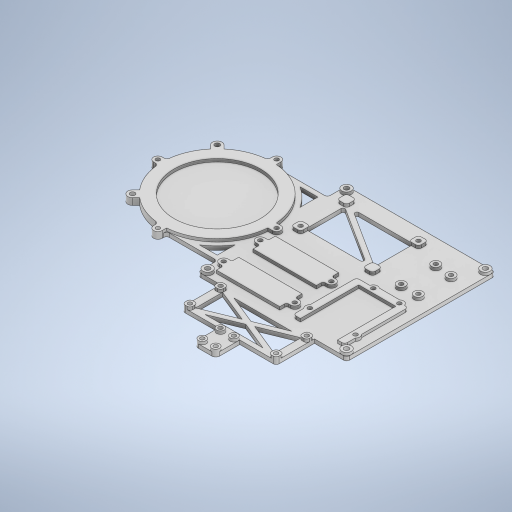
# Autodesk Inventor part: Base_BasePlate
Saved by Autodesk Inventor 2023 (Build 270158000, 158)
## iProperties
Created: 2025-02-05
Part Number: Base_BasePlate
Material: Generic
Document SubType Name: Modeling
Designer: Swoby
Density: 1 g/cm^3
Appearance: Default
Author: Swoby
Autodesk Inventor part; units mm, degrees
ref_plane "YZ Plane" through (0, 0, 0) normal (1, 0, 0) x (0, 1, 0)
ref_plane "XZ Plane" through (0, 0, 0) normal (0, 1, 0) x (-1, 0, 0)
ref_plane "XY Plane" through (0, 0, 0) normal (0, 0, 1) x (1, 0, 0)
sketch "Sketch1" plane through (0, 0, 0) normal (0, 1, 0) x (-1, 0, 0)
  line L0 (77.5, 77.5) -> (-77.5, 77.5)
  line L1 (-77.5, 77.5) -> (-77.5, -77.5)
  line L2 (-77.5, -77.5) -> (77.5, -77.5)
  line L3 (77.5, -77.5) -> (77.5, 77.5) construction
  line L4 (77.5, 77.5) -> (-77.5, -77.5) construction
  line L5 (-77.5, 77.5) -> (77.5, -77.5) construction
  line L6 (67.5, -9.5) -> (-17.6, -9.5) construction
  line L7 (-17.6, -9.5) -> (-17.6, -67.5) construction
  line L8 (-17.6, -67.5) -> (67.5, -67.5) construction
  line L9 (67.5, -67.5) -> (67.5, -9.5) construction
  line L10 (67.5, -9.5) -> (-17.6, -67.5) construction
  line L11 (-17.6, -9.5) -> (67.5, -67.5) construction
  circle A0 centre (62.5, -14.5) radius 2.1
  circle A1 centre (-12.6, -62.5) radius 2.1
  line L12 (57.5, -19.5) -> (67.5, -19.5)
  line L13 (67.5, -19.5) -> (67.5, -9.5)
  line L14 (67.5, -9.5) -> (57.5, -9.5)
  line L15 (57.5, -9.5) -> (57.5, -19.5)
  line L16 (57.5, -19.5) -> (67.5, -9.5) construction
  line L17 (67.5, -19.5) -> (57.5, -9.5) construction
  line L18 (-7.6, -57.5) -> (-17.6, -57.5)
  line L19 (-17.6, -57.5) -> (-17.6, -67.5)
  line L20 (-17.6, -67.5) -> (-7.6, -67.5)
  line L21 (-7.6, -67.5) -> (-7.6, -57.5)
  line L22 (-7.6, -57.5) -> (-17.6, -67.5) construction
  line L23 (-17.6, -57.5) -> (-7.6, -67.5) construction
  line L24 (-17.6, -9.5) -> (-7.6, -9.5)
  line L25 (-7.6, -9.5) -> (-7.6, -19.5)
  line L26 (-7.6, -19.5) -> (-17.6, -19.5)
  line L27 (-17.6, -19.5) -> (-17.6, -9.5)
  line L28 (67.5, -67.5) -> (57.5, -67.5)
  line L29 (57.5, -67.5) -> (57.5, -57.5)
  line L30 (57.5, -57.5) -> (67.5, -57.5)
  line L31 (67.5, -57.5) -> (67.5, -67.5)
  circle A2 centre (-42.6, -14.5) radius 2.1
  circle A3 centre (-42.6, -50.6) radius 2.1
  circle A4 centre (-60.5, -14.5) radius 2.1
  circle A5 centre (-60.5, -48.6) radius 2.1
  line L32 (-42.6, -14.5) -> (-42.6, -50.6) construction
  line L33 (-42.6, -14.5) -> (-60.5, -14.5) construction
  line L34 (-60.5, -14.5) -> (-60.5, -48.6) construction
  circle A6 centre (-42.6, -14.5) radius 4.5
  circle A7 centre (-42.6, -50.6) radius 4.5
  circle A8 centre (-60.5, -14.5) radius 4.5
  circle A9 centre (-60.5, -48.6) radius 4.5
  line L35 (-13.8, 69.5) -> (-67.5, 69.5)
  line L36 (-67.5, 69.5) -> (-67.5, 3.2)
  line L37 (-13.8, 3.2) -> (-13.8, 69.5)
  line L38 (-63.9, 3.2) -> (-61.4, 0.7)
  line L39 (-61.4, 0.7) -> (-29.8, 0.7)
  line L40 (-29.8, 0.7) -> (-27.3, 3.2)
  line L41 (-67.5, 3.2) -> (-63.9, 3.2)
  line L42 (-27.3, 3.2) -> (-13.8, 3.2)
  circle A10 centre (-64.5, 55.1) radius 2.1
  circle A11 centre (-16.8, 55.1) radius 2.1
  line L43 (77.5, 0) -> (77.5, 77.5) construction
  line L44 (77.5, 38.75) -> (5.2514, 38.75) construction
  line L45 (66.4, 69.5) -> (0.2, 69.5)
  line L46 (0.2, 69.5) -> (0.2, 62.35)
  line L47 (0.2, 46.2) -> (66.4, 46.2)
  line L48 (66.4, 46.2) -> (66.4, 69.5)
  circle A12 centre (-3.8, 57.85) radius 2.1
  circle A13 centre (70.4, 57.85) radius 2.1
  arc A14 (70.4, 53.35) -> (70.4, 62.35) centre (70.4, 57.85) ccw
  arc A15 (-3.8, 62.35) -> (-3.8, 53.35) centre (-3.8, 57.85) ccw
  line L49 (-3.8, 62.35) -> (0.2, 62.35)
  line L50 (-3.8, 53.35) -> (0.2, 53.35)
  line L51 (70.4, 62.35) -> (66.4, 62.35)
  line L52 (70.4, 53.35) -> (66.4, 53.35)
  line L53 (-3.8, 57.85) -> (70.4, 57.85) construction
  line L54 (33.3, 69.5) -> (33.3, 46.2) construction
  line L55 (66.4, 8) -> (0.2, 8)
  line L56 (0.2, 8) -> (0.2, 15.15)
  line L57 (0.2, 31.3) -> (66.4, 31.3)
  line L58 (66.4, 31.3) -> (66.4, 24.15)
  circle A16 centre (-3.8, 19.65) radius 2.1
  circle A17 centre (70.4, 19.65) radius 2.1
  arc A18 (70.4, 15.15) -> (70.4, 24.15) centre (70.4, 19.65) ccw
  arc A19 (-3.8, 24.15) -> (-3.8, 15.15) centre (-3.8, 19.65) ccw
  line L59 (-3.8, 15.15) -> (0.2, 15.15)
  line L60 (-3.8, 24.15) -> (0.2, 24.15)
  line L61 (70.4, 15.15) -> (66.4, 15.15)
  line L62 (70.4, 24.15) -> (66.4, 24.15)
  line L63 (-3.8, 19.65) -> (70.4, 19.65) construction
  line L64 (33.3, 8) -> (33.3, 31.3) construction
  circle A20 centre (-32, 4.1) radius 2.1
  circle A21 centre (-59.2, 4.1) radius 2.1
  line L65 (-32, 4.1) -> (-59.2, 4.1) construction
  line L66 (54, 117.5) -> (-44, 117.5)
  line L67 (-44, 117.5) -> (-44, 77.5)
  line L68 (-44, 77.5) -> (54, 77.5) construction
  line L69 (54, 77.5) -> (54, 117.5)
  line L70 (54, 117.5) -> (-44, 77.5) construction
  line L71 (-44, 117.5) -> (54, 77.5) construction
  line L72 (35.1344, 112.5) -> (-25.1344, 112.5)
  line L73 (-25.1344, 112.5) -> (5, 100.2002)
  line L74 (5, 100.2002) -> (35.1344, 112.5)
  line L75 (46, 111.5345) -> (11.6156, 97.5)
  line L76 (11.6156, 97.5) -> (46, 83.4655)
  line L77 (46, 83.4655) -> (46, 111.5345)
  line L78 (-36, 111.5345) -> (-1.6156, 97.5)
  line L79 (-1.6156, 97.5) -> (-36, 83.4655)
  line L80 (-36, 83.4655) -> (-36, 111.5345)
  line L81 (5, 94.7998) -> (-25.1344, 82.5)
  line L82 (-25.1344, 82.5) -> (35.1344, 82.5)
  line L83 (35.1344, 82.5) -> (5, 94.7998)
  line L84 (-40, 113.5) -> (50, 113.5) construction
  line L85 (50, 113.5) -> (50, 81.5) construction
  line L86 (50, 81.5) -> (-40, 81.5) construction
  line L87 (-40, 81.5) -> (-40, 113.5) construction
  line L88 (-40, 113.5) -> (50, 81.5) construction
  line L89 (50, 113.5) -> (-40, 81.5) construction
  circle A22 centre (50, 113.5) radius 2.1
  circle A23 centre (50, 81.5) radius 2.1
  circle A24 centre (-40, 113.5) radius 2.1
  circle A25 centre (-40, 81.5) radius 2.1
  line L90 (46, 109.5) -> (54, 109.5)
  line L91 (54, 109.5) -> (54, 117.5)
  line L92 (54, 117.5) -> (46, 117.5)
  line L93 (46, 117.5) -> (46, 109.5)
  line L94 (46, 109.5) -> (54, 117.5) construction
  line L95 (54, 109.5) -> (46, 117.5) construction
  line L96 (46, 85.5) -> (54, 85.5)
  line L97 (54, 85.5) -> (54, 77.5)
  line L98 (54, 77.5) -> (46, 77.5)
  line L99 (46, 77.5) -> (46, 85.5)
  line L100 (46, 85.5) -> (54, 77.5) construction
  line L101 (54, 85.5) -> (46, 77.5) construction
  line L102 (-36, 85.5) -> (-44, 85.5)
  line L103 (-44, 85.5) -> (-44, 77.5)
  line L104 (-44, 77.5) -> (-36, 77.5)
  line L105 (-36, 77.5) -> (-36, 85.5)
  line L106 (-36, 85.5) -> (-44, 77.5) construction
  line L107 (-44, 85.5) -> (-36, 77.5) construction
  line L108 (-36, 109.5) -> (-44, 109.5)
  line L109 (-44, 109.5) -> (-44, 117.5)
  line L110 (-44, 117.5) -> (-36, 117.5)
  line L111 (-36, 117.5) -> (-36, 109.5)
  line L112 (-36, 109.5) -> (-44, 117.5) construction
  line L113 (-44, 109.5) -> (-36, 117.5) construction
  circle A26 centre (135, 0) radius 45
  line L114 (135, 0) -> (77.5, 0) construction
  circle A27 centre (135, 0) radius 57.5
  line L115 (135, 57.5) -> (130.5, 57.5) construction
  line L116 (135, -57.5) -> (130.5, -57.5) construction
  line L117 (101.0884, 52.5) -> (82.5, 52.5)
  line L118 (82.5, 52.5) -> (82.5, 33.9116)
  arc A28 (101.0884, 52.5) -> (82.5, 33.9116) centre (135, 0) ccw
  line L119 (101.0884, -52.5) -> (82.5, -52.5)
  line L120 (82.5, -52.5) -> (82.5, -33.9116)
  arc A29 (82.5, -33.9116) -> (101.0884, -52.5) centre (135, 0) ccw
  arc A30 (77.5, 0) -> (73, 4.5) centre (73, 0) ccw construction
  circle A31 centre (73, 0) radius 2.1
  line L121 (135, 0) -> (192.5, 0) construction
  line L122 (135, 57.5) -> (135, -57.5) construction
  arc A32 (197, -4.5) -> (197, 4.5) centre (197, 0) ccw
  circle A33 centre (197, 0) radius 2.1
  line L123 (197, 4.5) -> (192.3236, 4.5)
  line L124 (197, -4.5) -> (192.3236, -4.5)
  line L125 (73, 4.5) -> (77.6764, 4.5)
  line L126 (73, -4.5) -> (77.6764, -4.5)
  line L127 (77.5, 77.5) -> (77.5, 57.5)
  line L128 (77.5, -77.5) -> (77.5, -57.5)
  arc A34 (139.5, 62) -> (130.5, 62) centre (135, 62) ccw
  circle A35 centre (135, 62) radius 2.1
  line L129 (139.5, 62) -> (139.5, 57.3236)
  line L130 (130.5, 62) -> (130.5, 57.3236)
  arc A36 (130.5, -62) -> (139.5, -62) centre (135, -62) ccw
  circle A37 centre (135, -62) radius 2.1
  line L131 (130.5, -62) -> (130.5, -57.3236)
  line L132 (139.5, -62) -> (139.5, -57.3236)
  line L133 (5, 97.5) -> (5, 117.5) construction
  circle A38 centre (-16.8, 55.1) radius 4.5
  circle A39 centre (-64.5, 55.1) radius 4.5
  circle A40 centre (-32, 4.1) radius 4.5
  circle A41 centre (-59.2, 4.1) radius 4.5
  line L134 (-21.3, 69.5) -> (-21.3, 8.6)
  line L135 (-21.3, 8.6) -> (-60, 8.6)
  line L136 (-60, 8.6) -> (-60, 69.5)
  arc A42 (73, -4.5) -> (77.5, 0) centre (73, 0) ccw construction
  arc A43 (73, 4.5) -> (73, -4.5) centre (73, 0) ccw
  line L137 (130.5, 57.5) -> (77.5, 57.5)
  line L138 (130.5, -57.5) -> (77.5, -57.5)
  line L139 (66.4, 15.15) -> (66.4, 8)
  line L140 (66.4, 19.65) -> (66.4, 15.15) construction
  line L141 (66.4, 24.15) -> (66.4, 19.65) construction
  line L142 (0.2, 15.15) -> (0.2, 24.15) construction
  line L143 (0.2, 24.15) -> (0.2, 31.3)
  line L144 (0.2, 62.35) -> (0.2, 53.35) construction
  line L145 (0.2, 53.35) -> (0.2, 46.2)
  point P0 (0, 0)
  point P1 (24.95, -38.5)
  point P2 (-51.55, -14.5)
  point P3 (-77.5, 0)
  point P4 (66.4, 57.85)
  point P5 (33.3, 57.85)
  point P6 (-8.3, 57.85)
  point P7 (33.3, 19.65)
  point P8 (-8.3, 19.65)
  point P9 (-67.5, 58.4541)
  point P10 (-67.5, 51.7459)
  point P11 (-63.5116, 2.8116)
  point P12 (-56.2521, 0.7)
  point P13 (-34.9479, 0.7)
  point P14 (-27.6884, 2.8116)
  point P15 (-13.8, 51.7459)
  point P16 (-13.8, 58.4541)
  dimension "d99" = 115
  dimension "d0" = 155
  dimension "d1" = 155
  dimension "d2" = 85.1
  dimension "d3" = 58
  dimension "d5" = 10
  dimension "d6" = 4.2
  dimension "d7" = 4.2
  dimension "d8" = 5
  dimension "d9" = 5
  dimension "d10" = 5
  dimension "d11" = 5
  dimension "d14" = 10
  dimension "d15" = 10
  dimension "d16" = 10
  dimension "d17" = 10
  dimension "d18" = 10
  dimension "d21" = 4.2
  dimension "d22" = 4.2
  dimension "d23" = 4.2
  dimension "d24" = 4.2
  dimension "d25" = 17.9
  dimension "d26" = 17.9
  dimension "d27" = 25
  dimension "d28" = 5
  dimension "d29" = 36.1
  dimension "d30" = 34.1
  dimension "d31" = 9
  dimension "d32" = 9
  dimension "d33" = 9
  dimension "d34" = 9
  dimension "d35" = 66.3
  dimension "d36" = 53.7
  dimension "d39" = 10
  dimension "d40" = 31.6
  dimension "d43" = 13.5
  dimension "d44" = 135
  dimension "d45" = 135
  dimension "d46" = 2.5
  dimension "d47" = 3
  dimension "d48" = 14.4
  dimension "d49" = 4.2
  dimension "d50" = 4.2
  dimension "d51" = 3
  dimension "d52" = 14.4
  dimension "d53" = 4.2
  dimension "d54" = 4.2
  dimension "d55" = 9
  dimension "d56" = 9
  dimension "d58" = 66.2
  dimension "d59" = 74.2
  dimension "d62" = 23.3
  dimension "d63" = 14
  dimension "d64" = 4.2
  dimension "d65" = 4.2
  dimension "d66" = 27.2
  dimension "d67" = 3.4
  dimension "d68" = 8.3
  dimension "d72" = 8
  dimension "d73" = 40
  dimension "d74" = 98
  dimension "d75" = 23.5
  dimension "d76" = 5
  dimension "d78" = 2.5
  dimension "d80" = 2.5
  constraints: 292 end point, 48 parallel, 43 centre point, 32 perpendicular, 30 midpoint, 27 horizontal, 25 point on circle, 25 point on line, 24 symmetric about line, 21 coincident, 21 tangent, 8 vertical, 4 collinear, 20 other
  measures "d0" distance of L2.end L1.end
  measures "d1" distance of L1.end L0.end
  measures "d2" distance of L8.end L7.end
  measures "d3" distance of L7.end L6.end
  measures "d5" distance between parallel lines of L3 L9
  measures "d6" diameter of A0
  measures "d7" diameter of A1
  measures "d8" distance from line of L9 A0.centre
  measures "d9" distance from line of L6 A0.centre
  measures "d10" distance from line of L7 A1.centre
  measures "d11" distance from line of L8 A1.centre
  measures "d14" distance between parallel lines of L2 L8
  measures "d15" distance of L25.end L26.end
  measures "d16" distance of L24.end L25.end
  measures "d17" distance of L29.end L30.end
  measures "d18" distance of L28.end L29.end
  measures "d21" diameter of A2
  measures "d22" diameter of A3
  measures "d23" diameter of A4
  measures "d24" diameter of A5
  measures "d25" distance of L32.start L33.end
  measures "d26" horizontal distance of L34.end L32.end
  measures "d27" distance between parallel lines of L32 L7
  measures "d28" distance from line of point (-51.55, -14.5) L6
  measures "d29" distance of L32.start L32.end
  measures "d30" distance of L33.end L34.end
  measures "d31" diameter of A6
  measures "d32" diameter of A7
  measures "d33" diameter of A8
  measures "d34" diameter of A9
  measures "d35" distance of L35.end L36.end
  measures "d36" distance of L35.start L35.end
  measures "d39" distance between parallel lines of L1 L36
  measures "d40" distance of L38.end L39.end
  measures "d43" distance of L40.end L37.start
  measures "d44" angle of L40 L42
  measures "d45" angle of L41 L38
  measures "d46" distance between parallel lines of L41 L39
  measures "d47" distance from line of L36 A10.centre
  measures "d48" distance from line of L35 A10.centre
  measures "d49" diameter of A10
  measures "d50" diameter of A11
  measures "d51" distance from line of L37 A11.centre
  measures "d52" distance from line of L35 A11.centre
  measures "d53" diameter of A12
  measures "d54" diameter of A13
  measures "d55" diameter of A14
  measures "d56" diameter of A15
  measures "d58" distance of L45.start L45.end
  measures "d59" distance of L53.start L53.end
  measures "d62" distance of L47.end L45.start
  measures "d63" distance between parallel lines of L37 L46
  measures "d64" diameter of A20
  measures "d65" diameter of A21
  measures "d66" distance of L65.start L65.end
  measures "d67" distance between parallel lines of L39 L65
  measures "d68" distance from line of L36 L65.end
  measures "d72" distance between parallel lines of L0 L35
  measures "d73" distance of L66.end L67.end
  measures "d74" distance of L66.start L66.end
  measures "d75" distance between parallel lines of L69 L3
  measures "d76" distance between parallel lines of L72 L66
  measures "d78" distance between parallel lines of L70 L74
  measures "d80" distance between parallel lines of L71 L73
extrude "Extrusion1" add sketch "Sketch1" against normal blind 4 contours L127 L137 L130 A27 L125 A43 L126 L131 L138 L128 L2 L1 L0 | L0 L99 L77 L96 L69 | L0 L105 L79 L78 L111 L66 L93 L75 L76 L99 | L96 L77 L90 L69 | L130 A34 L129 A27 | L0 L67 L102 L80 L105 | L90 L77 L93 L66 L69 | A27 | A27 L126 A43 L125 | L67 L108 L80 L102 | L123 A32 L124 A27 | L67 L66 L111 L80 L108 | A27 L132 A36 L131 | A0 | A1 | L15 L14 L13 L12 | L21 L20 L19 L18 | L24 L25 L26 L27 | L28 L29 L30 L31 | A2 | A3 | A4 | A5 | A6 | A7 | A8 | A9 | L37 A38 L134 L35 | L134 L135 L136 L35 | A38 L37 | L37 A38 | L136 A39 L36 L35 | A38 L37 L42 L40 A40 L135 L134 | A39 L36 | L136 L135 A41 L38 L41 L36 A39 | L36 A39 | A40 L40 L39 | A40 L39 A41 L135 | A41 L39 L38 | L39 L40 A40 | L38 L39 A41 | A10 | A11 | L48 L47 L145 L50 A15 L49 L46 L45 | L51 A14 L52 L48 | A12 | L55 L56 L59 A19 L60 L143 L57 L58 L62 A18 L61 L139 | A16 | A17 | A20 | A21 | A23 | A25 | A26 | A31 | A33 | A35 | A37
extrude "Extrusion2" add sketch "Sketch1" along normal blind 3 contours L0 L99 L77 L96 L69 | L130 A34 L129 A27 | L0 L67 L102 L80 L105 | L90 L77 L93 L66 L69 | A27 | A27 L126 A43 L125 | L123 A32 L124 A27 | L67 L66 L111 L80 L108 | A27 L132 A36 L131 | L15 L14 L13 L12 | L21 L20 L19 L18 | L24 L25 L26 L27 | L28 L29 L30 L31 | A6 | A7 | A8 | A9 | L37 A38 L134 L35 | A38 L37 | L37 A38 | L136 A39 L36 L35 | A38 L37 L42 L40 A40 L135 L134 | A39 L36 | L136 L135 A41 L38 L41 L36 A39 | L36 A39 | A40 L40 L39 | A40 L39 A41 L135 | A41 L39 L38 | L39 L40 A40 | L38 L39 A41 | L48 L47 L145 L50 A15 L49 L46 L45 | L51 A14 L52 L48 | L55 L56 L59 A19 L60 L143 L57 L58 L62 A18 L61 L139
fillet "Fillet1" radius 2 8 edges at (-0.2, 1.5, 53.35) (-0.2, 1.5, 62.35) (-0.2, 1.5, 24.15) (-0.2, 1.5, 15.15) (-66.4, 1.5, 62.35) (-66.4, 1.5, 53.35) (-66.4, 1.5, 24.15) (-66.4, 1.5, 15.15)
extrude "Extrusion3" cut sketch "Sketch1" against normal through all contours A0 | A1 | A2 | A5 | A10 | A11 | A12 | A13 | A16 | A17 | A20 | A21 | A22 | A23 | A24 | A25 | A31 | A33 | A35 | A37
fillet "Fillet2" radius 3 50 edges at (44, 1.5, 109.5) (36, 1.5, 109.5) (36, 1.5, 117.5) (67.5, 1.5, 69.5) (44, 1.5, 85.5) (36, 1.5, 85.5) (36, 1.5, 77.5) (44, 1.5, 77.5) (-54, 1.5, 109.5) (-46, 1.5, 117.5) (-46, 1.5, 109.5) (-46, 1.5, 85.5) (-46, 1.5, 77.5) (-54, 1.5, 77.5) (-54, 1.5, 85.5) (67.5, 1.5, 3.2) (13.8, 1.5, 3.2) (13.8, 1.5, 69.5) (17.6, 1.5, -9.5) (7.6, 1.5, -9.5) (7.6, 1.5, -19.5) (17.6, 1.5, -19.5) (7.6, 1.5, -57.5) (7.6, 1.5, -67.5) (17.6, 1.5, -57.5) (17.6, 1.5, -67.5) (-67.5, 1.5, -9.5) (-67.5, 1.5, -19.5) (-57.5, 1.5, -9.5) (-57.5, 1.5, -19.5) (-67.5, 1.5, -67.5) (-67.5, 1.5, -57.5) (-57.5, 1.5, -57.5) (-57.5, 1.5, -67.5) (-130.5, -2, 57.5) (-77.5, -2, 57.5) (-77.5, -2, -57.5) (-130.5, -2, -57.5) (-139.5, -0.5, -57.3236) (-139.5, -2, 57.3236) (-139.5, 1.5, 57.3236) (-192.3236, -2, 4.5) (-192.3236, 1.5, 4.5) (-192.3236, -0.5, -4.5) (-54, -0.5, 117.5) (44, -0.5, 117.5) (-77.5, -2, 77.5) (-77.5, -2, -77.5) (77.5, -2, -77.5) (77.5, -2, 77.5)
sketch "Sketch2" plane through (0, 0, 0) normal (0, 1, 0) x (1, 0, 0)
  circle A0 centre (-62.5, 14.5) radius 2.1 projected
  circle A1 centre (12.6, 62.5) radius 2.1 projected
  line L0 (-62.5, 14.5) -> (5.7571, 14.5) construction
  line L1 (12.6, 18.1519) -> (12.6, 62.5) construction
  line L2 (12.6, 62.5) -> (-55.6571, 62.5) construction
  line L3 (-62.5, 58.8481) -> (-62.5, 14.5) construction
  line L4 (-59.4229, 60.5333) -> (6.8342, 18.1852) construction
  line L5 (-56.7342, 58.8148) -> (9.5229, 16.4667) construction
  arc A2 (-59.4229, 60.5333) -> (-62.5, 58.8481) centre (-60.5, 58.8481) ccw construction
  arc A3 (-55.6571, 62.5) -> (-56.7342, 58.8148) centre (-55.6571, 60.5) ccw construction
  arc A4 (5.7571, 14.5) -> (6.8342, 18.1852) centre (5.7571, 16.5) ccw
  arc A5 (9.5229, 16.4667) -> (12.6, 18.1519) centre (10.6, 18.1519) ccw
  line L6 (-57.542, 17) -> (-2.7965, 17)
  line L7 (-1.7194, 20.6852) -> (-56.9229, 55.9684)
  line L8 (-60, 54.2832) -> (-60, 19.458)
  line L9 (-47.1035, 60) -> (7.642, 60)
  line L10 (10.1, 57.542) -> (10.1, 22.7168)
  line L11 (7.0229, 21.0316) -> (-48.1806, 56.3148)
  arc A6 (-56.9229, 55.9684) -> (-60, 54.2832) centre (-58, 54.2832) ccw
  arc A7 (-2.7965, 17) -> (-1.7194, 20.6852) centre (-2.7965, 19) ccw
  arc A8 (7.0229, 21.0316) -> (10.1, 22.7168) centre (8.1, 22.7168) ccw
  arc A9 (-47.1035, 60) -> (-48.1806, 56.3148) centre (-47.1035, 58) ccw
  arc A10 (-57.5, 16.5) -> (-60.5, 19.5) centre (-60.5, 16.5) ccw projected
  arc A11 (7.6, 60.5) -> (10.6, 57.5) centre (10.6, 60.5) ccw projected
  point P0 (0, 0)
  point P1 (12.6, 14.5)
  point P2 (-62.5, 62.5)
  dimension "d115" = 2
  dimension "d116" = 2
  dimension "d117" = 2.5
  dimension "d118" = 2.5
  dimension "d119" = 2
  dimension "d120" = 2.5
  dimension "d121" = 2.5
  dimension "d122" = 2.5
  dimension "d123" = 2.5
  constraints: 24 end point, 20 point on circle, 16 tangent, 8 centre point, 8 point on line, 6 parallel, 5 equal radius, 1 horizontal, 1 perpendicular
  measures "d115" radius of A2
  measures "d116" radius of A3
  measures "d117" distance between parallel lines of L3 L8
  measures "d118" distance between parallel lines of L2 L9
  measures "d119" radius of A6
  measures "d120" distance between parallel lines of L5 L7
  measures "d121" distance between parallel lines of L11 L4
  measures "d122" distance between parallel lines of L0 L6
  measures "d123" distance between parallel lines of L1 L10
extrude "Extrusion5" cut sketch "Sketch2" against normal through all contours A10 L8 A6 L7 A7 L6 | L9 A11 L10 A8 L11 A9
sketch "Sketch3" plane through (0, 0, 0) normal (0, 1, 0) x (1, 0, 0)
  line L0 (-46, -83.4655) -> (-11.6156, -97.5) projected
  line L1 (-11.6156, -97.5) -> (-46, -111.5345) projected
  line L2 (-46, -111.5345) -> (-46, -83.4655) projected
  line L3 (36, -83.4655) -> (36, -111.5345) projected
  line L4 (36, -111.5345) -> (1.6156, -97.5) projected
  line L5 (1.6156, -97.5) -> (36, -83.4655) projected
  line L6 (-5, -94.7998) -> (-35.1344, -82.5) projected
  line L7 (-35.1344, -82.5) -> (25.1344, -82.5) projected
  line L8 (25.1344, -82.5) -> (-5, -94.7998) projected
  line L9 (-35.1344, -112.5) -> (-5, -100.2002) projected
  line L10 (-5, -100.2002) -> (25.1344, -112.5) projected
  line L11 (25.1344, -112.5) -> (-35.1344, -112.5) projected
  arc A0 (-49, -85.5) -> (-46, -82.5) centre (-49, -82.5) ccw projected
  line L12 (-49, -85.5) -> (-51, -85.5) projected
  arc A1 (-54, -82.5) -> (-51, -85.5) centre (-51, -82.5) ccw projected
  line L13 (-54, -82.5) -> (-54, -112.5) projected
  arc A2 (-51, -109.5) -> (-54, -112.5) centre (-51, -112.5) ccw projected
  line L14 (-51, -109.5) -> (-49, -109.5) projected
  arc A3 (-46, -112.5) -> (-49, -109.5) centre (-49, -112.5) ccw projected
  line L15 (-46, -112.5) -> (-46, -114.5) projected
  arc A4 (-49, -117.5) -> (-46, -114.5) centre (-49, -114.5) ccw projected
  line L16 (-49, -117.5) -> (39, -117.5) projected
  arc A5 (36, -114.5) -> (39, -117.5) centre (39, -114.5) ccw projected
  line L17 (36, -114.5) -> (36, -112.5) projected
  arc A6 (39, -109.5) -> (36, -112.5) centre (39, -112.5) ccw projected
  line L18 (39, -109.5) -> (41, -109.5) projected
  arc A7 (44, -112.5) -> (41, -109.5) centre (41, -112.5) ccw projected
  line L19 (44, -112.5) -> (44, -82.5) projected
  arc A8 (41, -85.5) -> (44, -82.5) centre (41, -82.5) ccw projected
  line L20 (41, -85.5) -> (39, -85.5) projected
  arc A9 (36, -82.5) -> (39, -85.5) centre (39, -82.5) ccw projected
  line L21 (36, -82.5) -> (36, -80.5) projected
  arc A10 (39, -77.5) -> (36, -80.5) centre (39, -80.5) ccw projected
  line L22 (39, -77.5) -> (41, -77.5) projected
  arc A11 (-77.6764, 4.5) -> (-130.5, 57.3236) centre (-135, 0) ccw projected
  arc A12 (-46, -80.5) -> (-49, -77.5) centre (-49, -80.5) ccw projected
  line L23 (-46, -80.5) -> (-46, -82.5) projected
  line L24 (-12, -119.6) -> (2, -119.6) construction
  line L25 (2, -119.6) -> (2, -138.6) construction
  line L26 (2, -138.6) -> (-12, -138.6) construction
  line L27 (-12, -138.6) -> (-12, -119.6) construction
  circle A13 centre (-12, -119.6) radius 2.1
  circle A14 centre (2, -119.6) radius 2.1
  circle A15 centre (-12, -138.6) radius 2.1
  circle A16 centre (2, -138.6) radius 2.1
  line L28 (-5, -100.2002) -> (-5, -119.6)
  line L29 (-16, -117.5) -> (-16, -138.6)
  line L30 (-12, -142.6) -> (2, -142.6)
  line L31 (6, -138.6) -> (6, -117.5)
  arc A17 (-16, -138.6) -> (-12, -142.6) centre (-12, -138.6) ccw
  arc A18 (2, -142.6) -> (6, -138.6) centre (2, -138.6) ccw
  circle A19 centre (-12, -119.6) radius 4
  circle A20 centre (-12, -138.6) radius 4
  circle A21 centre (2, -138.6) radius 4
  circle A22 centre (2, -119.6) radius 4
  arc A23 (44, -80.5) -> (41, -77.5) centre (41, -80.5) ccw projected
  line L32 (44, -80.5) -> (44, -77.5) projected
  line L33 (44, -77.5) -> (74.5, -77.5) projected
  line L34 (77.5, -74.5) -> (77.5, 74.5) projected
  line L35 (74.5, 77.5) -> (-74.5, 77.5) projected
  line L36 (-77.5, 74.5) -> (-77.5, 60.5) projected
  arc A24 (-80.5, 57.5) -> (-77.5, 60.5) centre (-80.5, 60.5) ccw projected
  line L37 (-80.5, 57.5) -> (-127.5, 57.5) projected
  arc A25 (-130.5, 60.5) -> (-127.5, 57.5) centre (-127.5, 60.5) ccw projected
  line L38 (-130.5, 60.5) -> (-130.5, 57.3236) projected
  line L39 (-130.5, -57.3236) -> (-130.5, -60.5) projected
  arc A26 (-127.5, -57.5) -> (-130.5, -60.5) centre (-127.5, -60.5) ccw projected
  line L40 (-127.5, -57.5) -> (-80.5, -57.5) projected
  arc A27 (-77.5, -60.5) -> (-80.5, -57.5) centre (-80.5, -60.5) ccw projected
  line L41 (-77.5, -60.5) -> (-77.5, -74.5) projected
  line L42 (-74.5, -77.5) -> (-54, -77.5) projected
  line L43 (-54, -77.5) -> (-54, -80.5) projected
  arc A28 (-51, -77.5) -> (-54, -80.5) centre (-51, -80.5) ccw projected
  line L44 (-51, -77.5) -> (-49, -77.5) projected
  line L45 (-77.6764, 4.5) -> (-73, 4.5) projected
  arc A29 (-73, -4.5) -> (-73, 4.5) centre (-73, 0) ccw projected
  line L46 (-73, -4.5) -> (-77.6764, -4.5) projected
  arc A30 (-130.5, -57.3236) -> (-77.6764, -4.5) centre (-135, 0) ccw projected
  arc A31 (74.5, -77.5) -> (77.5, -74.5) centre (74.5, -74.5) ccw projected
  arc A32 (77.5, 74.5) -> (74.5, 77.5) centre (74.5, 74.5) ccw projected
  arc A33 (-74.5, 77.5) -> (-77.5, 74.5) centre (-74.5, 74.5) ccw projected
  arc A34 (-77.5, -74.5) -> (-74.5, -77.5) centre (-74.5, -74.5) ccw projected
  point P0 (0, 0)
  point P1 (-16, -142.6)
  point P2 (6, -142.6)
  point P3 (2, -117.5)
  point P4 (-12, -117.5)
  point P5 (-15.4044, -117.5)
  point P6 (-8.5956, -117.5)
  point P7 (-1.4044, -117.5)
  point P8 (5.4044, -117.5)
  point P9 (2, -142.6)
  dimension "d132" = 14
  dimension "d133" = 19
  dimension "d134" = 4.2
  dimension "d135" = 4.2
  dimension "d136" = 4.2
  dimension "d137" = 4.2
  dimension "d139" = 2.1
  dimension "d141" = 4
  dimension "d142" = 4
  dimension "d143" = 4
  dimension "d146" = 4
  dimension "d147" = 8
  dimension "d148" = 8
  dimension "d149" = 8
  dimension "d150" = 8
  constraints: 16 end point, 10 centre point, 8 coincident, 6 point on line, 4 point on circle, 4 tangent, 3 parallel, 3 perpendicular, 2 horizontal, 1 equal radius, 1 midpoint
  measures "d132" distance of L24.start L24.end
  measures "d133" distance of L24.end L25.end
  measures "d134" diameter of A13
  measures "d135" diameter of A14
  measures "d136" diameter of A15
  measures "d137" diameter of A16
  measures "d139" distance between parallel lines of L24 L16
  measures "d141" distance between parallel lines of L31 L25
  measures "d142" distance between parallel lines of L30 L26
  measures "d143" distance between parallel lines of L29 L27
  measures "d146" radius of A17
  measures "d147" diameter of A19
  measures "d148" diameter of A20
  measures "d149" diameter of A21
  measures "d150" diameter of A22
extrude "Extrusion6" add sketch "Sketch3" against normal up to surface (4 mm away) contours L16 A19 L29 | L16 A19 | A19 L16 A22 L31 A21 L30 A20 L29 | A20 A17 | L16 A22 | A21 A18 | L16 L31 A22 picked at (-8.6721, -119.9191) picked at (5.3264, -119.9251)
extrude "Extrusion7" add sketch "Sketch3" along normal blind 3 contours A19 L16 | L16 A19 | A20 A17 | A22 L16 | L16 A22 | A21 A18
sketch "Sketch4" plane through (0, 0, 0) normal (0, 1, 0) x (1, 0, 0)
  line L0 (36, -83.4655) -> (36, -111.5345) projected
  line L1 (36, -111.5345) -> (1.6156, -97.5) projected
  line L2 (1.6156, -97.5) -> (36, -83.4655) projected
  arc A0 (-101.0884, -52.5) -> (-82.5, -33.9116) centre (-135, 0) ccw projected
  line L3 (-82.5, -33.9116) -> (-82.5, -52.5) projected
  line L4 (-82.5, -52.5) -> (-101.0884, -52.5) projected
  line L5 (-82.5, 52.5) -> (-82.5, 33.9116) projected
  arc A1 (-82.5, 33.9116) -> (-101.0884, 52.5) centre (-135, 0) ccw projected
  line L6 (-101.0884, 52.5) -> (-82.5, 52.5) projected
  line L7 (-35.1344, -112.5) -> (-5, -100.2002) projected
  line L8 (-5, -100.2002) -> (25.1344, -112.5) projected
  line L9 (25.1344, -112.5) -> (-35.1344, -112.5) projected
  line L10 (-5, -94.7998) -> (-35.1344, -82.5) projected
  line L11 (-35.1344, -82.5) -> (25.1344, -82.5) projected
  line L12 (25.1344, -82.5) -> (-5, -94.7998) projected
  circle A2 centre (60.5, 14.5) radius 4.5 projected
  circle A3 centre (42.6, 14.5) radius 4.5 projected
  line L13 (-60, 19.458) -> (-60, 54.2832) projected
  arc A4 (-56.9229, 55.9684) -> (-60, 54.2832) centre (-58, 54.2832) ccw projected
  line L14 (-56.9229, 55.9684) -> (-1.7194, 20.6852) projected
  arc A5 (-2.7965, 17) -> (-1.7194, 20.6852) centre (-2.7965, 19) ccw projected
  line L15 (-2.7965, 17) -> (-57.542, 17) projected
  arc A6 (-57.5, 16.5) -> (-57.542, 17) centre (-60.5, 16.5) ccw projected
  line L16 (-57.5, 16.5) -> (-57.5, 12.5) projected
  arc A7 (-60.5, 9.5) -> (-57.5, 12.5) centre (-60.5, 12.5) ccw projected
  line L17 (-60.5, 9.5) -> (-64.5, 9.5) projected
  arc A8 (-67.5, 12.5) -> (-64.5, 9.5) centre (-64.5, 12.5) ccw projected
  line L18 (-67.5, 12.5) -> (-67.5, 16.5) projected
  arc A9 (-64.5, 19.5) -> (-67.5, 16.5) centre (-64.5, 16.5) ccw projected
  line L19 (-64.5, 19.5) -> (-60.5, 19.5) projected
  arc A10 (-60, 19.458) -> (-60.5, 19.5) centre (-60.5, 16.5) ccw projected
  line L20 (-67.5, 60.5) -> (-67.5, 64.5) projected
  arc A11 (-64.5, 67.5) -> (-67.5, 64.5) centre (-64.5, 64.5) ccw projected
  line L21 (-64.5, 67.5) -> (-60.5, 67.5) projected
  arc A12 (-57.5, 64.5) -> (-60.5, 67.5) centre (-60.5, 64.5) ccw projected
  line L22 (-57.5, 64.5) -> (-57.5, 60.5) projected
  arc A13 (-60.5, 57.5) -> (-57.5, 60.5) centre (-60.5, 60.5) ccw projected
  line L23 (-60.5, 57.5) -> (-64.5, 57.5) projected
  arc A14 (-67.5, 60.5) -> (-64.5, 57.5) centre (-64.5, 60.5) ccw projected
  circle A15 centre (60.5, 48.6) radius 4.5 projected
  circle A16 centre (42.6, 50.6) radius 4.5 projected
  line L24 (17.6, 16.5) -> (17.6, 12.5) projected
  arc A17 (14.6, 9.5) -> (17.6, 12.5) centre (14.6, 12.5) ccw projected
  line L25 (14.6, 9.5) -> (10.6, 9.5) projected
  arc A18 (7.6, 12.5) -> (10.6, 9.5) centre (10.6, 12.5) ccw projected
  line L26 (7.6, 12.5) -> (7.6, 16.5) projected
  arc A19 (10.6, 19.5) -> (7.6, 16.5) centre (10.6, 16.5) ccw projected
  line L27 (10.6, 19.5) -> (14.6, 19.5) projected
  arc A20 (17.6, 16.5) -> (14.6, 19.5) centre (14.6, 16.5) ccw projected
  line L28 (10.1, 57.542) -> (10.1, 22.7168) projected
  arc A21 (7.0229, 21.0316) -> (10.1, 22.7168) centre (8.1, 22.7168) ccw projected
  line L29 (7.0229, 21.0316) -> (-48.1806, 56.3148) projected
  arc A22 (-47.1035, 60) -> (-48.1806, 56.3148) centre (-47.1035, 58) ccw projected
  line L30 (-47.1035, 60) -> (7.642, 60) projected
  arc A23 (7.6, 60.5) -> (7.642, 60) centre (10.6, 60.5) ccw projected
  line L31 (7.6, 60.5) -> (7.6, 64.5) projected
  arc A24 (10.6, 67.5) -> (7.6, 64.5) centre (10.6, 64.5) ccw projected
  line L32 (10.6, 67.5) -> (14.6, 67.5) projected
  arc A25 (17.6, 64.5) -> (14.6, 67.5) centre (14.6, 64.5) ccw projected
  line L33 (17.6, 64.5) -> (17.6, 60.5) projected
  arc A26 (14.6, 57.5) -> (17.6, 60.5) centre (14.6, 60.5) ccw projected
  line L34 (14.6, 57.5) -> (10.6, 57.5) projected
  arc A27 (10.1, 57.542) -> (10.6, 57.5) centre (10.6, 60.5) ccw projected
  line L35 (60, -69.5) -> (60, -8.6) projected
  line L36 (60, -8.6) -> (21.3, -8.6) projected
  line L37 (21.3, -8.6) -> (21.3, -69.5) projected
  line L38 (21.3, -69.5) -> (16.8, -69.5) projected
  arc A28 (13.8, -66.5) -> (16.8, -69.5) centre (16.8, -66.5) ccw projected
  line L39 (13.8, -66.5) -> (13.8, -58.4541) projected
  arc A29 (13.8, -51.7459) -> (13.8, -58.4541) centre (16.8, -55.1) ccw projected
  line L40 (13.8, -51.7459) -> (13.8, -6.2) projected
  arc A30 (16.8, -3.2) -> (13.8, -6.2) centre (16.8, -6.2) ccw projected
  line L41 (16.8, -3.2) -> (27.3, -3.2) projected
  line L42 (27.3, -3.2) -> (27.6884, -2.8116) projected
  arc A31 (34.9479, -0.7) -> (27.6884, -2.8116) centre (32, -4.1) ccw projected
  line L43 (34.9479, -0.7) -> (56.2521, -0.7) projected
  arc A32 (63.5116, -2.8116) -> (56.2521, -0.7) centre (59.2, -4.1) ccw projected
  line L44 (63.5116, -2.8116) -> (63.9, -3.2) projected
  line L45 (63.9, -3.2) -> (64.5, -3.2) projected
  arc A33 (67.5, -6.2) -> (64.5, -3.2) centre (64.5, -6.2) ccw projected
  line L46 (67.5, -6.2) -> (67.5, -51.7459) projected
  arc A34 (67.5, -58.4541) -> (67.5, -51.7459) centre (64.5, -55.1) ccw projected
  line L47 (67.5, -58.4541) -> (67.5, -66.5) projected
  arc A35 (64.5, -69.5) -> (67.5, -66.5) centre (64.5, -66.5) ccw projected
  line L48 (64.5, -69.5) -> (60, -69.5) projected
  arc A36 (-68.4, -53.35) -> (-66.4, -51.35) centre (-68.4, -51.35) ccw projected
  line L49 (-66.4, -51.35) -> (-66.4, -46.2) projected
  line L50 (-66.4, -46.2) -> (-0.2, -46.2) projected
  line L51 (-0.2, -46.2) -> (-0.2, -51.35) projected
  arc A37 (-0.2, -51.35) -> (1.8, -53.35) centre (1.8, -51.35) ccw projected
  line L52 (1.8, -53.35) -> (3.8, -53.35) projected
  arc A38 (3.8, -62.35) -> (3.8, -53.35) centre (3.8, -57.85) ccw projected
  line L53 (3.8, -62.35) -> (1.8, -62.35) projected
  arc A39 (1.8, -62.35) -> (-0.2, -64.35) centre (1.8, -64.35) ccw projected
  line L54 (-0.2, -64.35) -> (-0.2, -69.5) projected
  line L55 (-0.2, -69.5) -> (-66.4, -69.5) projected
  line L56 (-66.4, -69.5) -> (-66.4, -64.35) projected
  arc A40 (-66.4, -64.35) -> (-68.4, -62.35) centre (-68.4, -64.35) ccw projected
  line L57 (-68.4, -62.35) -> (-70.4, -62.35) projected
  arc A41 (-70.4, -53.35) -> (-70.4, -62.35) centre (-70.4, -57.85) ccw projected
  line L58 (-70.4, -53.35) -> (-68.4, -53.35) projected
  arc A42 (-68.4, -15.15) -> (-66.4, -13.15) centre (-68.4, -13.15) ccw projected
  line L59 (-66.4, -13.15) -> (-66.4, -8) projected
  line L60 (-66.4, -8) -> (-0.2, -8) projected
  line L61 (-0.2, -8) -> (-0.2, -13.15) projected
  arc A43 (-0.2, -13.15) -> (1.8, -15.15) centre (1.8, -13.15) ccw projected
  line L62 (1.8, -15.15) -> (3.8, -15.15) projected
  arc A44 (3.8, -24.15) -> (3.8, -15.15) centre (3.8, -19.65) ccw projected
  line L63 (3.8, -24.15) -> (1.8, -24.15) projected
  arc A45 (1.8, -24.15) -> (-0.2, -26.15) centre (1.8, -26.15) ccw projected
  line L64 (-0.2, -26.15) -> (-0.2, -31.3) projected
  line L65 (-0.2, -31.3) -> (-66.4, -31.3) projected
  line L66 (-66.4, -31.3) -> (-66.4, -26.15) projected
  arc A46 (-66.4, -26.15) -> (-68.4, -24.15) centre (-68.4, -26.15) ccw projected
  line L67 (-68.4, -24.15) -> (-70.4, -24.15) projected
  arc A47 (-70.4, -15.15) -> (-70.4, -24.15) centre (-70.4, -19.65) ccw projected
  line L68 (-70.4, -15.15) -> (-68.4, -15.15) projected
  line L69 (-46, -83.4655) -> (-11.6156, -97.5) projected
  line L70 (-11.6156, -97.5) -> (-46, -111.5345) projected
  line L71 (-46, -111.5345) -> (-46, -83.4655) projected
  arc A48 (-12, -142.6) -> (-16, -138.6) centre (-12, -138.6) ccw projected
  line L72 (-12, -142.6) -> (2, -142.6) projected
  arc A49 (6, -138.6) -> (2, -142.6) centre (2, -138.6) ccw projected
  line L73 (6, -138.6) -> (6, -119.6) projected
  circle A50 centre (2, -119.6) radius 4 projected
  line L74 (6, -119.6) -> (6, -117.5) projected
  line L75 (6, -117.5) -> (39, -117.5) projected
  arc A51 (36, -114.5) -> (39, -117.5) centre (39, -114.5) ccw projected
  line L76 (36, -114.5) -> (36, -112.5) projected
  arc A52 (39, -109.5) -> (36, -112.5) centre (39, -112.5) ccw projected
  line L77 (39, -109.5) -> (41, -109.5) projected
  arc A53 (44, -112.5) -> (41, -109.5) centre (41, -112.5) ccw projected
  line L78 (44, -112.5) -> (44, -82.5) projected
  arc A54 (41, -85.5) -> (44, -82.5) centre (41, -82.5) ccw projected
  line L79 (41, -85.5) -> (39, -85.5) projected
  arc A55 (36, -82.5) -> (39, -85.5) centre (39, -82.5) ccw projected
  line L80 (36, -82.5) -> (36, -80.5) projected
  arc A56 (39, -77.5) -> (36, -80.5) centre (39, -80.5) ccw projected
  line L81 (39, -77.5) -> (41, -77.5) projected
  arc A57 (44, -80.5) -> (41, -77.5) centre (41, -80.5) ccw projected
  line L82 (44, -80.5) -> (44, -77.5) projected
  line L83 (44, -77.5) -> (74.5, -77.5) projected
  arc A58 (74.5, -77.5) -> (77.5, -74.5) centre (74.5, -74.5) ccw projected
  line L84 (77.5, -74.5) -> (77.5, 74.5) projected
  arc A59 (77.5, 74.5) -> (74.5, 77.5) centre (74.5, 74.5) ccw projected
  line L85 (74.5, 77.5) -> (-74.5, 77.5) projected
  arc A60 (-74.5, 77.5) -> (-77.5, 74.5) centre (-74.5, 74.5) ccw projected
  line L86 (-77.5, 74.5) -> (-77.5, 60.5) projected
  arc A61 (-80.5, 57.5) -> (-77.5, 60.5) centre (-80.5, 60.5) ccw projected
  line L87 (-80.5, 57.5) -> (-127.5, 57.5) projected
  arc A62 (-130.5, 60.5) -> (-127.5, 57.5) centre (-127.5, 60.5) ccw projected
  line L88 (-130.5, 60.5) -> (-130.5, 57.3236) projected
  arc A63 (-77.6764, 4.5) -> (-130.5, 57.3236) centre (-135, 0) ccw projected
  line L89 (-77.6764, 4.5) -> (-73, 4.5) projected
  arc A64 (-73, -4.5) -> (-73, 4.5) centre (-73, 0) ccw projected
  line L90 (-73, -4.5) -> (-77.6764, -4.5) projected
  arc A65 (-130.5, -57.3236) -> (-77.6764, -4.5) centre (-135, 0) ccw projected
  line L91 (-130.5, -57.3236) -> (-130.5, -60.5) projected
  arc A66 (-127.5, -57.5) -> (-130.5, -60.5) centre (-127.5, -60.5) ccw projected
  line L92 (-127.5, -57.5) -> (-80.5, -57.5) projected
  arc A67 (-77.5, -60.5) -> (-80.5, -57.5) centre (-80.5, -60.5) ccw projected
  line L93 (-77.5, -60.5) -> (-77.5, -74.5) projected
  arc A68 (-77.5, -74.5) -> (-74.5, -77.5) centre (-74.5, -74.5) ccw projected
  line L94 (-74.5, -77.5) -> (-54, -77.5) projected
  line L95 (-54, -77.5) -> (-54, -80.5) projected
  arc A69 (-51, -77.5) -> (-54, -80.5) centre (-51, -80.5) ccw projected
  line L96 (-51, -77.5) -> (-49, -77.5) projected
  arc A70 (-46, -80.5) -> (-49, -77.5) centre (-49, -80.5) ccw projected
  line L97 (-46, -80.5) -> (-46, -82.5) projected
  arc A71 (-49, -85.5) -> (-46, -82.5) centre (-49, -82.5) ccw projected
  line L98 (-49, -85.5) -> (-51, -85.5) projected
  arc A72 (-54, -82.5) -> (-51, -85.5) centre (-51, -82.5) ccw projected
  line L99 (-54, -82.5) -> (-54, -112.5) projected
  arc A73 (-51, -109.5) -> (-54, -112.5) centre (-51, -112.5) ccw projected
  line L100 (-51, -109.5) -> (-49, -109.5) projected
  arc A74 (-46, -112.5) -> (-49, -109.5) centre (-49, -112.5) ccw projected
  line L101 (-46, -112.5) -> (-46, -114.5) projected
  arc A75 (-49, -117.5) -> (-46, -114.5) centre (-49, -114.5) ccw projected
  line L102 (-49, -117.5) -> (-16, -117.5) projected
  line L103 (-16, -117.5) -> (-16, -119.6) projected
  circle A76 centre (-12, -119.6) radius 4 projected
  line L104 (-16, -119.6) -> (-16, -138.6) projected
  arc A77 (-77.6764, 4.5) -> (-130.5, 57.3236) centre (-135, 0) ccw projected
  line L105 (-130.5, 57.3236) -> (-130.5, 62) projected
  arc A78 (-130.5, 62) -> (-139.5, 62) centre (-135, 62) ccw projected
  line L106 (-139.5, 62) -> (-139.5, 60.0333) projected
  arc A79 (-142.1281, 57.0565) -> (-139.5, 60.0333) centre (-142.5, 60.0333) ccw projected
  arc A80 (-142.1281, 57.0565) -> (-192.0565, 7.1281) centre (-135, 0) ccw projected
  arc A81 (-195.0333, 4.5) -> (-192.0565, 7.1281) centre (-195.0333, 7.5) ccw projected
  line L107 (-195.0333, 4.5) -> (-197, 4.5) projected
  arc A82 (-197, 4.5) -> (-197, -4.5) centre (-197, 0) ccw projected
  line L108 (-197, -4.5) -> (-195.0333, -4.5) projected
  arc A83 (-192.0565, -7.1281) -> (-195.0333, -4.5) centre (-195.0333, -7.5) ccw projected
  arc A84 (-192.0565, -7.1281) -> (-142.1281, -57.0565) centre (-135, 0) ccw projected
  arc A85 (-139.5, -60.0333) -> (-142.1281, -57.0565) centre (-142.5, -60.0333) ccw projected
  line L109 (-139.5, -60.0333) -> (-139.5, -62) projected
  arc A86 (-139.5, -62) -> (-130.5, -62) centre (-135, -62) ccw projected
  line L110 (-130.5, -62) -> (-130.5, -57.3236) projected
  arc A87 (-130.5, -57.3236) -> (-77.6764, -4.5) centre (-135, 0) ccw projected
  line L111 (-77.6764, -4.5) -> (-73, -4.5) projected
  arc A88 (-73, -4.5) -> (-73, 4.5) centre (-73, 0) ccw projected
  line L112 (-73, 4.5) -> (-77.6764, 4.5) projected
  circle A89 centre (-135, 0) radius 45 projected
  circle A90 centre (-73, 0) radius 2.1 projected
  circle A91 centre (-135, 62) radius 2.1 projected
  circle A92 centre (-197, 0) radius 2.1 projected
  circle A93 centre (-135, -62) radius 2.1 projected
  circle A94 centre (-135, 0) radius 45 projected
  line L113 (-135, 0) -> (-179.1942, 44.1942) construction
  line L114 (-135, 0) -> (-179.1942, -44.1942) construction
  line L115 (-197, 0) -> (-135, 0)
  circle A95 centre (-179.1942, 44.1942) radius 2.5
  arc A96 (-175.6586, 47.7297) -> (-182.7297, 40.6586) centre (-179.1942, 44.1942) ccw
  circle A97 centre (-179.1942, -44.1942) radius 2.5
  arc A98 (-182.7297, -40.6586) -> (-175.6586, -47.7297) centre (-179.1942, -44.1942) ccw
  line L116 (-182.7297, -40.6586) -> (-179.0402, -36.9691)
  line L117 (-175.6586, -47.7297) -> (-171.9691, -44.0402)
  arc A99 (-175.6586, -40.6586) -> (-182.7297, -40.6586) centre (-179.1942, -44.1942) ccw construction
  arc A100 (-175.6586, -47.7297) -> (-175.6586, -40.6586) centre (-179.1942, -44.1942) ccw construction
  line L118 (-182.7297, 40.6586) -> (-179.0402, 36.9691)
  line L119 (-175.6586, 47.7297) -> (-171.9691, 44.0402)
  arc A101 (-175.6586, 40.6586) -> (-175.6586, 47.7297) centre (-179.1942, 44.1942) ccw construction
  arc A102 (-182.7297, 40.6586) -> (-175.6586, 40.6586) centre (-179.1942, 44.1942) ccw construction
  line L120 (-74.5, 74.5) -> (74.5, -74.5) construction
  line L121 (-74.5, -74.5) -> (74.5, 74.5) construction
  line L122 (-72.5, -72.5) -> (72.5, -72.5) construction
  line L123 (72.5, -72.5) -> (72.5, 72.5) construction
  line L124 (72.5, 72.5) -> (-72.5, 72.5) construction
  line L125 (-72.5, 72.5) -> (-72.5, -72.5) construction
  line L126 (-72.5, -72.5) -> (72.5, 72.5) construction
  line L127 (72.5, -72.5) -> (-72.5, 72.5) construction
  circle A103 centre (-72.5, 72.5) radius 2.5
  circle A104 centre (72.5, 72.5) radius 2.5
  circle A105 centre (-72.5, -72.5) radius 2.5
  circle A106 centre (72.5, -72.5) radius 2.5
  circle A107 centre (-72.5, 72.5) radius 5
  circle A108 centre (72.5, 72.5) radius 5
  circle A109 centre (72.5, -72.5) radius 5
  circle A110 centre (-72.5, -72.5) radius 5
  point P0 (0, 0)
  dimension "d157" = 45
  dimension "d158" = 45
  dimension "d159" = 5
  dimension "d160" = 10
  dimension "d161" = 5
  dimension "d162" = 10
  dimension "d163" = 145
  dimension "d164" = 5
  dimension "d165" = 5
  dimension "d166" = 5
  dimension "d167" = 5
  dimension "d168" = 10
  dimension "d169" = 10
  dimension "d170" = 10
  dimension "d171" = 10
  constraints: 30 end point, 16 centre point, 16 point on circle, 11 coincident, 11 tangent, 6 parallel, 3 point on line, 2 horizontal, 2 horizontal alignment, 2 midpoint, 2 perpendicular
  measures "d157" angle of L113 L115
  measures "d158" angle of L114 L115
  measures "d159" diameter of A95
  measures "d160" diameter of A96
  measures "d161" diameter of A97
  measures "d162" diameter of A98
  measures "d163" distance of L123.end L124.end
  measures "d164" diameter of A103
  measures "d165" diameter of A104
  measures "d166" diameter of A105
  measures "d167" diameter of A106
  measures "d168" diameter of A107
  measures "d169" diameter of A108
  measures "d170" diameter of A109
  measures "d171" diameter of A110
extrude "Extrusion8 - Uchyceni" add sketch "Sketch4" along normal blind 3 and the other way blind 4 contours A110 | A109 | A108 | A107 | L117 A98 L116 A84 | A80 L118 A96 L119
extrude "Extrusion9 - Uchyceni" cut sketch "Sketch4" against normal through all contours A103 | A104 | A105 | A106
body "Solid1"
